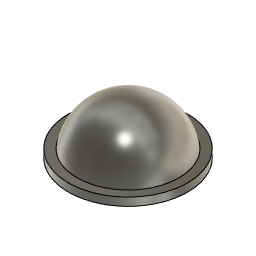
POP_Endcap (Autodesk Fusion 360 design; units mm, degrees)
Autodesk Fusion 360 part; units mm, degrees
sketch "Sketch1" plane through (0, 0, 0) normal (0, 1, 0) x (1, 0, 0)
  line L0 (-36, 0) -> (40, 0) construction
  arc A0 (-32, 0) -> (0, -32) centre (0, 0) ccw
  arc A1 (-22, 0) -> (0, -22) centre (0, 0) ccw
  line L1 (0, -32) -> (0, -22)
  line L2 (-22, 0) -> (-32, 0)
  dimension "d3" = 22
  dimension "d4" = 32
  constraint coincident A0.centre A1.centre
  constraint horizontal L0
  constraint coincident L0 A0.start
  constraint coincident L0 A1.start
  measures "d3" radius of A1
  measures "d4" radius of A0
revolve "Revolve1" add sketch "Sketch1" angle 360 about axis through (0, 0, 1.75) along (0, 0, 1)
sketch "Sketch2" plane through (0, 0, 0) normal (0, 0, -1) x (1, 0, 0)
  circle A0 centre (0, 0) radius 32
  circle A1 centre (0, 0) radius 22
  circle A2 centre (0, 0) radius 25.1968
  circle A3 centre (0, 0) radius 28.956
  dimension "d6" = 50.3936
  dimension "d7" = 57.912
  constraint coincident A0.centre A1.centre
  measures "d6" diameter of A2
  measures "d7" diameter of A3
extrude "Extrude1" cut sketch "Sketch2" against normal blind 2.921 contours A3
sketch "Sketch3" plane through (0, 0, 0) normal (0, 0, -1) x (1, 0, 0)
  circle A0 centre (0, 0) radius 32
  circle A1 centre (0, 0) radius 28.956
  circle A2 centre (0, 0) radius 37
  dimension "d10" = 74
  constraint coincident A0.centre A1.centre
  measures "d10" diameter of A2
extrude "Extrude2" add sketch "Sketch3" against normal blind 5 contours A0 | A2
fillet "Fillet1" radius 0.05 2 edges at (-23.4917, 9.1116, 0) (-26.9965, -10.4709, 0)
